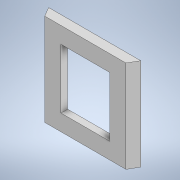
# Autodesk Inventor part: SatelliteSideWallSensor_v2
Saved by Autodesk Inventor 2020 (Build 240168000, 168)
## iProperties
Created: 2020-03-05
Part Number: SatelliteSideWallSensor_v2
Material: Generic
Document SubType Name: Modeling
Designer: WANG
Density: 1 g/cm^3
Appearance: Default
Author: WANG
Autodesk Inventor part; units mm, degrees
ref_plane "YZ Plane" through (0, 0, 0) normal (1, 0, 0) x (0, 1, 0)
ref_plane "XZ Plane" through (0, 0, 0) normal (0, 1, 0) x (-1, 0, 0)
ref_plane "XY Plane" through (0, 0, 0) normal (0, 0, 1) x (1, 0, 0)
sketch "Sketch1" plane through (0, 0, 0) normal (0, 1, 0) x (-1, 0, 0)
  line L0 (-107.95, 0) -> (-53.975, 93.4874)
  line L1 (-53.975, 93.4874) -> (53.975, 93.4874)
  line L2 (53.975, 93.4874) -> (107.95, 0)
  line L3 (107.95, 0) -> (53.975, -93.4874)
  line L4 (53.975, -93.4874) -> (-53.975, -93.4874)
  line L5 (-53.975, -93.4874) -> (-107.95, 0)
  line L6 (-95.25, 0.0344) -> (-47.5952, 82.5062)
  line L7 (-47.5952, 82.5062) -> (47.6548, 82.4717)
  line L8 (47.6548, 82.4717) -> (95.25, -0.0344)
  line L9 (95.25, -0.0344) -> (47.5952, -82.5062)
  line L10 (47.5952, -82.5062) -> (-47.6548, -82.4717)
  line L11 (-47.6548, -82.4717) -> (-95.25, 0.0344)
  line L12 (53.975, -93.4874) -> (47.5952, -82.5062)
  line L13 (-53.975, -93.4874) -> (-47.6548, -82.4717)
  point P0 (0, 0)
  point P1 (0, 0)
  point P2 (0, 0)
  point P3 (0, 0)
  dimension "d0" = 215.9
  dimension "d1" = 12.7
  constraints: 28 end point, 2 coincident, 26 other
  measures "d0" distance of L0.start L2.end
  measures "d1" distance of L0.start L6.start
extrude "Extrusion1" add sketch "Sketch1" along normal blind 107.95 contours L13 L10 L12 L4
sketch "Sketch2" plane through (47.6548, 0, -82.4717) normal (-0.0003616, 0, 0.9999999) x (0.9999999, 0, 0.0003616)
  line L0 (-95.2501, 0) -> (-95.2501, 107.95) projected
  line L1 (-95.2501, 107.95) -> (0, 107.95) projected
  line L2 (-95.2501, 0) -> (0, 0) projected
  line L3 (0, 0) -> (0, 107.95) projected
  line L4 (-76.2001, 88.9) -> (-19.05, 88.9)
  line L5 (-19.05, 88.9) -> (-19.05, 19.05)
  line L6 (-19.05, 19.05) -> (-76.2001, 19.05)
  line L7 (-76.2001, 19.05) -> (-76.2001, 88.9)
  point P0 (-47.625, 0)
  dimension "d4" = 19.05
  dimension "d5" = 19.05
  dimension "d6" = 19.05
  dimension "d7" = 19.05
  constraints: 8 end point, 2 parallel, 1 horizontal, 1 perpendicular
  measures "d4" distance from line of L0 L4.start
  measures "d5" distance from line of L1 L4.start
  measures "d6" distance from line of L2 L5.end
  measures "d7" distance from line of L3 L5.end
extrude "Extrusion2" cut sketch "Sketch2" against normal up to surface (11.0157 mm away) contours L4 L5 L6 L7
sketch "Sketch3" plane through (53.975, 0, -93.4874) normal (0, 0, -1) x (-1, 0, 0)
  line L0 (0, 107.95) -> (107.95, 107.95) projected
  line L1 (0, 0) -> (0, 107.95) projected
  line L2 (25.3662, 88.9) -> (82.5162, 88.9) projected
  line L3 (25.3662, 19.05) -> (25.3662, 88.9) projected
  line L4 (82.5162, 88.9) -> (82.5162, 19.05) projected
  line L5 (82.5162, 19.05) -> (25.3662, 19.05) projected
  line L6 (19.0162, 95.25) -> (88.8662, 95.25)
  line L7 (88.8662, 95.25) -> (88.8662, 12.7)
  line L8 (88.8662, 12.7) -> (19.0162, 12.7)
  line L9 (19.0162, 12.7) -> (19.0162, 95.25)
  point P0 (53.975, 0)
  dimension "d12" = 6.35
  dimension "d13" = 6.35
  dimension "d14" = 6.35
  dimension "d15" = 6.35
  constraints: 8 end point, 2 parallel, 1 horizontal, 1 perpendicular
  measures "d12" distance from line of L2 L6.start
  measures "d13" distance from line of L3 L6.start
  measures "d14" distance from line of L4 L7.end
  measures "d15" distance from line of L5 L7.end
extrude "Extrusion3" cut sketch "Sketch3" against normal blind 3.175 contours L2 L4 L5 L3 | L6 L7 L8 L9
equation "\"d6\" = d5"
equation "\"d7\" = d4"
equation "\"d14\" = d13"
equation "\"d15\" = d12"
body "Solid1"
